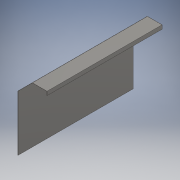
# Autodesk Inventor part: Front Panel
Saved by Autodesk Inventor 2018 (Build 220112000, 112)
## iProperties
Created: 2018-08-09
Part Number: Front Panel
Material: Steel
Document SubType Name: Modeling
Designer: P301319
Density: 7.85 g/cm^3
Appearance: Stainless - Brushed
Author: P301319
Autodesk Inventor part; units mm, degrees
ref_plane "YZ Plane" through (0, 0, 0) normal (1, 0, 0) x (0, 1, 0)
ref_plane "XZ Plane" through (0, 0, 0) normal (0, 1, 0) x (-1, 0, 0)
ref_plane "XY Plane" through (0, 0, 0) normal (0, 0, 1) x (1, 0, 0)
sketch "Sketch1" plane through (0, 0, 0) normal (0, 0, 1) x (1, 0, 0)
  line L0 (150, 800) -> (304, 800)
  line L1 (150, 800) -> (0, 650)
  line L2 (150, 800) -> (1016.5277, 800) construction
  line L3 (304, 800) -> (304, 760)
  line L4 (0, 650) -> (0, 70)
  line L5 (1.6, 70) -> (1.6, 649.3373)
  line L6 (1.6, 649.3373) -> (150.6627, 798.4)
  line L7 (150.6627, 798.4) -> (302.4, 798.4)
  line L8 (302.4, 798.4) -> (302.4, 760)
  line L9 (1.6, 70) -> (0, 70)
  line L10 (304, 760) -> (302.4, 760)
  point P0 (0, 0)
  dimension "d0" = 154
  dimension "d1" = 800
  dimension "d2" = 135
  dimension "d4" = 40
  dimension "d8" = 150
  dimension "d9" = 580
  dimension "d10" = 70
  dimension "d12" = 1.6
  constraints: 22 end point, 4 horizontal, 2 vertical, 3 other
  measures "d0" distance of L0.start L0.end
  measures "d1" distance from line of point (0, 0) L0
  measures "d2" angle of L1 L2
  measures "d4" distance of L0.end L3.end
  measures "d8" horizontal distance of point (0, 0) L0.start
  measures "d9" distance of L1.end L4.end
  measures "d10" distance of point (0, 0) L4.end
  measures "d12" distance between parallel lines of L1 L6
extrude "Extrusion1" add sketch "Sketch1" along normal blind 1200
body "Solid1"
